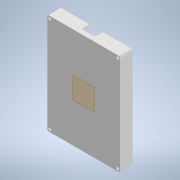
# Autodesk Inventor part: Bottom_lid
Saved by Autodesk Inventor 2022 (Build 260153000, 153)
## iProperties
Created: 2021-01-26
Part Number: Bottom_lid
Material: Generic
Document SubType Name: Modeling
Designer: simen
Density: 1 g/cm^3
Appearance: Default
Author: simen
## iProperties of the stored document Bottom_lid_3DPrint.ipt
Created: 2021-12-09
Part Number: Bottom_lid_3DPrint
Material: Generic
Document SubType Name: Modeling
Designer: simen
Density: 1 g/cm^3
Appearance: Default
Author: simen
Autodesk Inventor part; units mm, degrees
ref_plane "YZ Plane" through (0, 0, 0) normal (1, 0, 0) x (0, 1, 0)
ref_plane "XZ Plane" through (0, 0, 0) normal (0, 1, 0) x (-1, 0, 0)
ref_plane "XY Plane" through (0, 0, 0) normal (0, 0, 1) x (1, 0, 0)
ref_plane "Work Plane4" through (0, 0, 0) normal (0, 0, 1) x (1, 0, 0)
sketch "Sketch1" plane through (0, 0, 0) normal (0, 0, 1) x (1, 0, 0)
  line L0 (37, 49) -> (37, -49) projected
  arc A0 (37, 49) -> (35, 51) centre (35, 49) ccw projected
  line L1 (-35, 51) -> (35, 51) projected
  line L2 (-37, -49) -> (-37, 49) projected
  arc A1 (-35, 51) -> (-37, 49) centre (-35, 49) ccw projected
  arc A2 (-37, -49) -> (-35, -51) centre (-35, -49) ccw projected
  line L3 (35, -51) -> (-35, -51) projected
  arc A3 (35, -51) -> (37, -49) centre (35, -49) ccw projected
  arc A4 (36.8, 49) -> (35, 50.8) centre (35, 49) ccw
  line L4 (36.8, 49) -> (36.8, -49)
  arc A5 (35, -50.8) -> (36.8, -49) centre (35, -49) ccw
  line L5 (35, -50.8) -> (-35, -50.8)
  arc A6 (-36.8, -49) -> (-35, -50.8) centre (-35, -49) ccw
  line L6 (-36.8, -49) -> (-36.8, 49)
  arc A7 (-35, 50.8) -> (-36.8, 49) centre (-35, 49) ccw
  line L7 (-35, 50.8) -> (35, 50.8)
  point P0 (0, 0)
  point P1 (34.3, 48.3)
  point P2 (-33, 42)
  dimension "d0" = 0.2
  constraints: 8 end point, 8 point on circle, 4 centre point, 7 other
  measures "d0" distance between parallel lines of L1 L7
extrude "Extrusion1" add sketch "Sketch1" against normal blind 2 contours L4 A5 L5 A6 L6 A7 L7 A4
sketch "Sketch4" plane through (0, 0, 0) normal (0, 0, 1) x (1, 0, 0)
  line L0 (36.8, -49) -> (36.8, 49) projected
  arc A0 (36.8, 49) -> (35, 50.8) centre (35, 49) ccw projected
  line L1 (35, 50.8) -> (-35, 50.8) projected
  arc A1 (-35, 50.8) -> (-36.8, 49) centre (-35, 49) ccw projected
  line L2 (-36.8, 49) -> (-36.8, -49) projected
  arc A2 (-36.8, -49) -> (-35, -50.8) centre (-35, -49) ccw projected
  line L3 (-35, -50.8) -> (35, -50.8) projected
  arc A3 (35, -50.8) -> (36.8, -49) centre (35, -49) ccw projected
  circle A4 centre (34.3, 48.3) radius 1.4
  circle A5 centre (34.3, -48.3) radius 1.4
  circle A6 centre (-34.3, -48.3) radius 1.4
  circle A7 centre (-34.3, 48.3) radius 1.4
  point P0 (0, 0)
  dimension "d22" = 2.8
  dimension "d23" = 2.8
  dimension "d24" = 2.8
  dimension "d25" = 2.8
  dimension "d59" = 2.5
  dimension "d60" = 2.5
  dimension "d62" = 2.5
  dimension "d63" = 2.5
  dimension "d64" = 2.5
  dimension "d65" = 2.5
  dimension "d66" = 2.5
  dimension "d67" = 2.5
  constraints: 4 centre point, 3 coincident
  measures "d22" diameter of A4
  measures "d23" diameter of A5
  measures "d24" diameter of A6
  measures "d25" diameter of A7
  measures "d59" distance from line of L0 A4.centre
  measures "d60" distance from line of A4.centre L1
  measures "d62" distance from line of L1 A7.centre
  measures "d63" distance from line of L2 A7.centre
  measures "d64" distance from line of L3 A6.centre
  measures "d65" distance from line of L2 A6.centre
  measures "d66" distance from line of L0 A5.centre
  measures "d67" distance from line of L3 A5.centre
extrude "Extrusion3" cut sketch "Sketch4" against normal blind 10 contours A4 | A5 | A6 | A7
ref_plane "Work Plane5" through (0, 0, -2) normal (0, 0, -1) x (-1, 0, 0)
sketch "Sketch5" plane through (0, 0, -2) normal (0, 0, -1) x (-1, 0, 0)
  line L0 (-34.8, 48.8) -> (34.8, 48.8)
  line L1 (34.8, 48.8) -> (34.8, -48.8)
  line L2 (34.8, -48.8) -> (-34.8, -48.8)
  line L3 (-34.8, -48.8) -> (-34.8, 48.8)
  circle A0 centre (34.3, 48.3) radius 1.4 projected
  circle A1 centre (34.3, -48.3) radius 1.4 projected
  circle A2 centre (-34.3, -48.3) radius 1.4 projected
  circle A3 centre (-34.3, 48.3) radius 1.4 projected
  circle A4 centre (-34.3, 48.3) radius 2.9
  circle A5 centre (-34.3, -48.3) radius 2.9
  circle A6 centre (34.3, -48.3) radius 2.9
  circle A7 centre (34.3, 48.3) radius 2.9
  circle A8 centre (34.3, -48.3) radius 1.4 projected
  circle A9 centre (34.3, 48.3) radius 1.4 projected
  circle A10 centre (-34.3, -48.3) radius 1.4 projected
  circle A11 centre (-34.3, 48.3) radius 1.4 projected
  line L4 (-36.8, 49) -> (-36.8, -49) projected
  arc A12 (-36.8, -49) -> (-35, -50.8) centre (-35, -49) ccw projected
  line L5 (-35, -50.8) -> (35, -50.8) projected
  arc A13 (35, -50.8) -> (36.8, -49) centre (35, -49) ccw projected
  line L6 (36.8, -49) -> (36.8, 49) projected
  arc A14 (36.8, 49) -> (35, 50.8) centre (35, 49) ccw projected
  line L7 (35, 50.8) -> (-35, 50.8) projected
  arc A15 (-35, 50.8) -> (-36.8, 49) centre (-35, 49) ccw projected
  point P0 (0, 0)
  point P1 (-31.4434, 48.8)
  point P2 (31.4434, 48.8)
  point P3 (34.8, 45.4434)
  point P4 (34.8, -45.4434)
  point P5 (31.4434, -48.8)
  point P6 (-31.4434, -48.8)
  point P7 (-34.8, -45.4434)
  point P8 (-34.8, 45.4434)
  dimension "d68" = 1.5
  dimension "d69" = 1.5
  dimension "d70" = 1.5
  dimension "d71" = 1.5
  constraints: 8 end point, 4 centre point
  measures "d68" radial gap between concentric circles of A3 A4
  measures "d69" radial gap between concentric circles of A2 A5
  measures "d70" radial gap between concentric circles of A1 A6
  measures "d71" radial gap between concentric circles of A0 A7
extrude "Extrusion4" add sketch "Sketch5" along normal blind 10.7 contours L3 A3 L0 | L0 A3 L3 | A3 L3 A4 L4 A15 L7 L0 | L0 A4 L3 A3 | A4 L7 A7 L0 | L3 A5 L4 A4 | A7 L7 A14 L6 L1 A0 L0 | L0 A0 L1 A7 | A5 L2 A2 L3 | L3 A2 L2 A5 L5 A12 L4 | A0 L1 L0 | L0 L1 A0 | A7 L6 A6 L1 | A2 L2 L3 | L3 L2 A2 | A6 L6 A13 L5 L2 A1 L1 | L1 A1 L2 A6 | L2 A6 L5 A5 | A1 L2 L1 | L1 L2 A1
sketch "Sketch6" plane through (-34.3, 48.3, -2) normal (0, 0, 1) x (1, 0, 0)
  circle A0 centre (68.6, 0) radius 1.4 projected
  circle A1 centre (0, 0) radius 1.4 projected
  circle A2 centre (0, -96.6) radius 1.4 projected
  circle A3 centre (68.6, -96.6) radius 1.4 projected
  circle A4 centre (68.6, 0) radius 0.8
  circle A5 centre (0, 0) radius 0.8
  circle A6 centre (0, -96.6) radius 0.8
  circle A7 centre (68.6, -96.6) radius 0.8
  point P0 (34.3, -48.3)
  dimension "d47" = 1.6
  dimension "d48" = 1.6
  dimension "d49" = 1.6
  dimension "d50" = 1.6
  constraints: 4 centre point, 4 coincident
  measures "d47" diameter of A4
  measures "d48" diameter of A5
  measures "d49" diameter of A6
  measures "d50" diameter of A7
extrude "Extrusion5" cut sketch "Sketch6" against normal through all contours A4 | A5 | A6 | A7
sketch "Sketch7" plane through (-34.3, 48.3, -2) normal (0, 0, 1) x (1, 0, 0)
  circle A0 centre (0, 0) radius 1.4 projected
  circle A1 centre (0, -96.6) radius 1.4 projected
  circle A2 centre (68.6, -96.6) radius 1.4 projected
  circle A3 centre (68.6, 0) radius 1.4 projected
  point P0 (34.3, -48.3)
extrude "Extrusion6" cut sketch "Sketch7" against normal blind 7.9
sketch "Sketch8" plane through (0, 0, -12.7) normal (0, 0, -1) x (-1, 0, 0)
  circle A0 centre (-34.3, -48.3) radius 0.8 projected
  circle A1 centre (-34.3, 48.3) radius 0.8 projected
  circle A2 centre (34.3, -48.3) radius 0.8 projected
  circle A3 centre (34.3, 48.3) radius 0.8 projected
  arc A4 (-36.8, -49) -> (-35, -50.8) centre (-35, -49) ccw projected
  line L0 (-35, -50.8) -> (35, -50.8) projected
  arc A5 (35, -50.8) -> (36.8, -49) centre (35, -49) ccw projected
  line L1 (36.8, -49) -> (36.8, 49) projected
  arc A6 (36.8, 49) -> (35, 50.8) centre (35, 49) ccw projected
  line L2 (35, 50.8) -> (-35, 50.8) projected
  arc A7 (-35, 50.8) -> (-36.8, 49) centre (-35, 49) ccw projected
  line L3 (-36.8, 49) -> (-36.8, -49) projected
  line L4 (-31.4434, 48.8) -> (31.4434, 48.8) projected
  arc A8 (31.4434, 48.8) -> (34.8, 45.4434) centre (34.3, 48.3) ccw projected
  line L5 (34.8, 45.4434) -> (34.8, -45.4434) projected
  arc A9 (34.8, -45.4434) -> (31.4434, -48.8) centre (34.3, -48.3) ccw projected
  line L6 (31.4434, -48.8) -> (-31.4434, -48.8) projected
  arc A10 (-31.4434, -48.8) -> (-34.8, -45.4434) centre (-34.3, -48.3) ccw projected
  line L7 (-34.8, -45.4434) -> (-34.8, 45.4434) projected
  arc A11 (-34.8, 45.4434) -> (-31.4434, 48.8) centre (-34.3, 48.3) ccw projected
  line L8 (34.8, 45.4434) -> (34.8, -45.4434) projected
  line L9 (36.8, 10.8) -> (34.8, 10.8)
  line L10 (34.8, 10.8) -> (34.8, -10.8)
  line L11 (34.8, -10.8) -> (36.8, -10.8)
  line L12 (36.8, -10.8) -> (36.8, 10.8)
  line L13 (35, 50.8) -> (-35, 50.8) projected
  line L14 (-31.4434, 48.8) -> (31.4434, 48.8) projected
  line L15 (-6.8, 50.8) -> (6.8, 50.8)
  line L16 (6.8, 50.8) -> (6.8, 48.8)
  line L17 (6.8, 48.8) -> (-6.8, 48.8)
  line L18 (-6.8, 48.8) -> (-6.8, 50.8)
  point P0 (0, 0)
  dimension "d74" = 40
  dimension "d75" = 40
  dimension "d76" = 30
  dimension "d77" = 30
  constraints: 16 end point, 4 parallel, 4 point on line, 2 horizontal, 2 perpendicular
  measures "d74" distance between parallel lines of L0 L11
  measures "d75" distance between parallel lines of L2 L9
  measures "d76" distance between parallel lines of L1 L16
  measures "d77" distance between parallel lines of L3 L18
extrude "Extrusion7" cut sketch "Sketch8" against normal blind 8 contours L2 L16 L4 L18 | L11 L5 L9 L1
fillet "Fillet3" radius 2 4 edges at (-35.8, -10.8, -4.7) (-35.8, 10.8, -4.7) (-6.8, 49.8, -4.7) (6.8, 49.8, -4.7)
body "Solid1"
